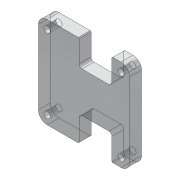
# Autodesk Inventor part: QUIKS_SINGLE_COVER
Saved by Autodesk Inventor 2019.4 (Build 234330000, 330)
## iProperties
Created: 2019-12-27
Part Number: QUIKS_SINGLE_COVER
Material: 一般
Document SubType Name: Modeling
Designer: y6tada
Density: 1 g/cm^3
Appearance: クリア
Author: y6tada
Autodesk Inventor part; units mm, degrees
ref_plane "YZ Plane" through (0, 0, 0) normal (1, 0, 0) x (0, 1, 0)
ref_plane "XZ Plane" through (0, 0, 0) normal (0, 1, 0) x (-1, 0, 0)
ref_plane "XY Plane" through (0, 0, 0) normal (0, 0, 1) x (1, 0, 0)
sketch "スケッチ1" plane through (0, 0, 0) normal (0, 0, 1) x (1, 0, 0)
  line L0 (12.35, 15.25) -> (9.34, 15.25)
  line L1 (-15.25, 12.35) -> (-15.25, -12.35)
  line L2 (-12.35, -15.25) -> (-1.66, -15.25)
  line L3 (15.25, -12.35) -> (15.25, 12.35)
  line L4 (-0.66, 6.75) -> (8.34, 6.75)
  line L5 (9.34, 7.75) -> (9.34, 15.25)
  line L6 (-0.66, -6.75) -> (8.34, -6.75)
  line L7 (9.34, -7.75) -> (9.34, -15.25)
  line L8 (9.34, 15.25) -> (-1.66, 15.25) construction
  line L9 (-1.66, 15.25) -> (-12.35, 15.25)
  line L10 (9.34, -15.25) -> (12.35, -15.25)
  line L11 (-1.66, -15.25) -> (9.34, -15.25) construction
  line L12 (-1.66, 15.25) -> (-1.66, 7.75)
  line L13 (-1.66, -15.25) -> (-1.66, -7.75)
  arc A0 (15.25, 12.35) -> (12.35, 15.25) centre (12.35, 12.35) ccw
  arc A1 (12.35, -15.25) -> (15.25, -12.35) centre (12.35, -12.35) ccw
  arc A2 (-15.25, -12.35) -> (-12.35, -15.25) centre (-12.35, -12.35) ccw
  arc A3 (-12.35, 15.25) -> (-15.25, 12.35) centre (-12.35, 12.35) ccw
  arc A4 (-1.66, 7.75) -> (-0.66, 6.75) centre (-0.66, 7.75) ccw
  arc A5 (8.34, 6.75) -> (9.34, 7.75) centre (8.34, 7.75) ccw
  arc A6 (9.34, -7.75) -> (8.34, -6.75) centre (8.34, -7.75) ccw
  arc A7 (-0.66, -6.75) -> (-1.66, -7.75) centre (-0.66, -7.75) ccw
  line L14 (0, 0) -> (0, -35.1049) construction
  line L15 (0, 0) -> (30.4007, 0) construction
  line L16 (3.84, -9) -> (3.84, -1.2529) construction
  arc A8 (15.35, 12.35) -> (12.35, 15.35) centre (12.35, 12.35) ccw construction
  dimension "d0" = 2.9
  dimension "d1" = 1
  dimension "d14" = 8.5
  dimension "d15" = 11
  dimension "d16" = 3.84
  dimension "d17" = 8.5
  dimension "d21" = 3
  constraints: 34 end point, 18 point on circle, 16 tangent, 12 parallel, 9 centre point, 6 equal radius, 6 horizontal, 4 coincident, 3 perpendicular, 3 vertical, 2 collinear, 1 concentric, 7 other
  measures "d0" radius of A0
  measures "d1" radius of A4
  measures "d14" distance between parallel lines of L2 L6
  measures "d15" distance between parallel lines of L13 L7
  measures "d16" distance between parallel lines of L14 L16
  measures "d17" distance between parallel lines of L9 L4
  measures "d21" radius of A8
extrude "押し出し1" add sketch "スケッチ1" along normal blind 4
hole "穴1" at (12.35, 12.35, 0) at (12.35, -12.35, 0) at (-12.35, -12.35, 0) at (-12.35, 12.35, 0) direction (0, 0, 1) diameter 2.1 end through all
chamfer "面取り1" distance 0.25 angle 45 4 edges at (9.34, 15.25, 2) (-1.66, 15.25, 2) (-1.66, -15.25, 2) (9.34, -15.25, 2)
